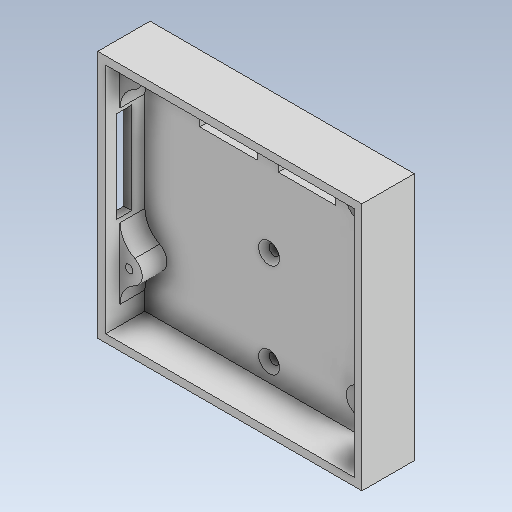
# Autodesk Inventor part: 10-06-004 carcasa spate
Saved by Autodesk Inventor 2020 (Build 240168000, 168)
## iProperties
Created: 2019-11-09
Part Number: 10-06-004 carcasa spate
Material: Generic
Document SubType Name: Modeling
Designer: iuliu
Density: 1 g/cm^3
Appearance: Default
Mass: 65.159 g
Surface Area: 324.526 cm^2
Volume: 65.159 cm^3
Description: Carcasa spate Display
Author: iuliu
Subject: 039
Autodesk Inventor part; units mm, degrees
ref_plane "YZ Plane" through (0, 0, 0) normal (1, 0, 0) x (0, 1, 0)
ref_plane "XZ Plane" through (0, 0, 0) normal (0, 1, 0) x (-1, 0, 0)
ref_plane "XY Plane" through (0, 0, 0) normal (0, 0, 1) x (1, 0, 0)
sketch "Sketch1" plane through (0, 0, 0) normal (0, 0, 1) x (1, 0, 0)
  line L0 (-50.5, 47.5) -> (50.5, 47.5)
  line L1 (50.5, 47.5) -> (50.5, -47.5)
  line L2 (50.5, -47.5) -> (-50.5, -47.5)
  line L3 (-50.5, -47.5) -> (-50.5, 47.5)
  point P0 (0, 0)
  point P1 (0, 47.5)
  point P2 (-50.5, 0)
  dimension "d0" = 95
  dimension "d1" = 101
  constraints: 8 end point, 2 midpoint, 2 parallel, 1 horizontal, 1 horizontal alignment, 1 perpendicular, 1 vertical alignment
  measures "d0" distance of L2.end L0.start
  measures "d1" distance of L0.start L0.end
extrude "Extrusion1" add sketch "Sketch1" along normal blind 20
sketch "Sketch2" plane through (0, 0, 20) normal (0, 0, 1) x (1, 0, 0)
  line L0 (-50.5, 47.5) -> (-50.5, -47.5) projected
  line L1 (-50.5, -47.5) -> (50.5, -47.5) projected
  line L2 (50.5, -47.5) -> (50.5, 47.5) projected
  line L3 (50.5, 47.5) -> (-50.5, 47.5) projected
  line L4 (-47.5, 44.5) -> (-47.5, -44.5)
  line L5 (-47.5, -44.5) -> (47.5, -44.5)
  line L6 (47.5, -44.5) -> (47.5, 44.5)
  line L7 (47.5, 44.5) -> (-47.5, 44.5)
  point P0 (0, 0)
  dimension "d4" = 3
  constraints: 8 end point, 3 other
  measures "d4" distance between parallel lines of L7 L3
extrude "Extrusion2" cut sketch "Sketch2" against normal blind 15 contours L7 L6 L5 L4
sketch "Sketch3" plane through (0, 0, 5) normal (0, 0, 1) x (1, 0, 0)
  line L0 (-25.5, 37) -> (-5.5, 37) projected
  line L1 (-25.5, 28) -> (-25.5, 37) projected
  line L2 (-5.5, 28) -> (-25.5, 28) projected
  line L3 (-5.5, 37) -> (-5.5, 28) projected
  line L4 (4.5, 37) -> (24.5, 37) projected
  line L5 (4.5, 28) -> (4.5, 37) projected
  line L6 (24.5, 28) -> (4.5, 28) projected
  line L7 (24.5, 37) -> (24.5, 28) projected
  line L8 (-4.5, 38) -> (-26.5, 38)
  line L9 (-26.5, 38) -> (-26.5, 27)
  line L10 (-26.5, 27) -> (-4.5, 27)
  line L11 (-4.5, 27) -> (-4.5, 38)
  line L12 (25.5, 38) -> (3.5, 38)
  line L13 (3.5, 38) -> (3.5, 27)
  line L14 (3.5, 27) -> (25.5, 27)
  line L15 (25.5, 27) -> (25.5, 38)
  point P0 (0, 0)
  dimension "d7" = 1
  dimension "d8" = 1
  constraints: 16 end point, 6 other
  measures "d7" distance between parallel lines of L0 L8
  measures "d8" distance between parallel lines of L4 L12
extrude "Extrusion3" cut sketch "Sketch3" against normal through all contours L0 L3 L2 L1 | L4 L7 L6 L5 | L11 L10 L9 L8 | L15 L14 L13 L12
sketch "Sketch4" plane through (0, 0, 5) normal (0, 0, 1) x (1, 0, 0)
  circle A0 centre (-44, -24) radius 1.5 projected
  circle A1 centre (44, -24) radius 1.5 projected
  circle A2 centre (44, 41) radius 1.5 projected
  circle A3 centre (-44, 41) radius 1.5 projected
  circle A4 centre (-44, -24) radius 5
  circle A5 centre (44, -24) radius 5
  circle A6 centre (-44, 41) radius 5
  circle A7 centre (44, 41) radius 5
  point P0 (0, 0)
  dimension "d11" = 10
  dimension "d12" = 10
  dimension "d13" = 10
  dimension "d14" = 10
  constraints: 4 centre point, 4 coincident
  measures "d11" diameter of A4
  measures "d12" diameter of A5
  measures "d13" diameter of A6
  measures "d14" diameter of A7
extrude "Extrusion4" add sketch "Sketch4" along normal blind 9.5
fillet "Fillet1" radius 10 8 edges at (-47.5, -27.5707, 9.75) (-47.5, -20.4293, 9.75) (47.5, -20.4293, 9.75) (47.5, -27.5707, 9.75) (47.5, 37.4293, 9.75) (40.4293, 44.5, 9.75) (-40.4293, 44.5, 9.75) (-47.5, 37.4293, 9.75)
sketch "Sketch7" plane through (-50.5, -47.5, 0) normal (-1, 0, 0) x (0, 0, 1)
  line L0 (10, 73.75) -> (16, 73.75)
  line L1 (16, 73.75) -> (16, 38.75)
  line L2 (16, 38.75) -> (10, 38.75)
  line L3 (10, 38.75) -> (10, 73.75)
  line L4 (20, 95) -> (20, 0) projected
  line L5 (0, 0) -> (20, 0) projected
  point P0 (0, 47.5)
  dimension "d18" = 6
  dimension "d19" = 35
  dimension "d20" = 4
  dimension "d21" = 38.75
  constraints: 8 end point, 2 parallel, 1 horizontal, 1 perpendicular
  measures "d18" distance of L0.start L0.end
  measures "d19" distance of L2.end L0.start
  measures "d20" distance between parallel lines of L4 L1
  measures "d21" distance between parallel lines of L5 L2
extrude "Extrusion5" cut sketch "Sketch7" against normal up to surface (3 mm away)
sketch "Sketch9" plane through (0, 0, 5) normal (0, 0, 1) x (1, 0, 0)
  circle A0 centre (0, -1.5) radius 2.5 construction
  circle A1 centre (0, -37.5) radius 2.5 construction
  point P0 (0, 0)
hole "Hole2" at (0, -1.5, 5) at (0, -37.5, 5) direction (0, 0, -1) diameter 4 end through all countersink diameter 8 countersink angle 90
body "Solid1"
